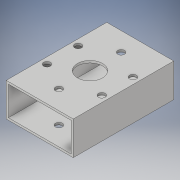
# Autodesk Inventor part: hub attachment
Saved by Autodesk Inventor 2018 (Build 220112000, 112)
## iProperties
Created: 2019-01-30
Part Number: hub attachment
Material: Generic
Document SubType Name: Modeling
Designer: s-4008082
Density: 1 g/cm^3
Appearance: Default
Author: s-4008082
Autodesk Inventor part; units mm, degrees
ref_plane "YZ Plane" through (0, 0, 0) normal (1, 0, 0) x (0, 1, 0)
ref_plane "XZ Plane" through (0, 0, 0) normal (0, 1, 0) x (-1, 0, 0)
ref_plane "XY Plane" through (0, 0, 0) normal (0, 0, 1) x (1, 0, 0)
sketch "Sketch1" plane through (0, 0, 0) normal (0, 0, 1) x (1, 0, 0)
  line L0 (0, 0) -> (50.8, 0)
  line L1 (50.8, 0) -> (50.8, 25.4)
  line L2 (50.8, 25.4) -> (0, 25.4)
  line L3 (0, 25.4) -> (0, 0)
  line L4 (49.149, 23.749) -> (1.651, 23.749)
  line L5 (1.651, 23.749) -> (1.651, 1.651)
  line L6 (1.651, 1.651) -> (49.149, 1.651)
  line L7 (49.149, 1.651) -> (49.149, 23.749)
  line L8 (49.149, 23.749) -> (1.651, 1.651) construction
  line L9 (1.651, 23.749) -> (49.149, 1.651) construction
  point P0 (25.4, 12.7)
  dimension "d0" = 1.651
  dimension "d1" = 25.4
  dimension "d2" = 50.8
  dimension "d3" = 1.651
  dimension "d4" = 1.651
  dimension "d5" = 1.651
  constraints: 20 end point, 4 parallel, 2 horizontal, 2 midpoint, 2 perpendicular
  measures "d0" distance between parallel lines of L2 L4
  measures "d1" distance of L0.end L1.end
  measures "d2" distance of L1.end L2.end
  measures "d3" distance between parallel lines of L1 L7
  measures "d4" distance between parallel lines of L0 L6
  measures "d5" distance between parallel lines of L3 L5
extrude "Extrusion1" add sketch "Sketch1" along normal blind 76.2
sketch "Sketch2" plane through (0, 25.4, 0) normal (0, 1, 0) x (1, 0, 0)
  circle A0 centre (25.4, -38.1) radius 9.525
  line L0 (50.8, 0) -> (50.8, -76.2) projected
  line L1 (50.8, -76.2) -> (0, -76.2) projected
  point P0 (0, 0)
  dimension "d8" = 19.05
  dimension "d9" = 25.4
  dimension "d10" = 38.1
  constraints: 1 centre point
  measures "d8" diameter of A0
  measures "d9" distance from line of L0 A0.centre
  measures "d10" distance from line of L1 A0.centre
extrude "Extrusion2" cut sketch "Sketch2" against normal blind 76.2
sketch "Sketch4" plane through (0, 25.4, 0) normal (0, 1, 0) x (1, 0, 0)
  circle A0 centre (25.1665, -14.2875) radius 2.5797
  circle A1 centre (25.4, -38.1) radius 9.525 projected
  circle A2 centre (25.4, -38.1) radius 23.8136 construction
  circle A3 centre (4.661, -26.396) radius 2.5797
  circle A4 centre (4.8945, -50.2085) radius 2.5797
  circle A5 centre (25.6335, -61.9125) radius 2.5797
  circle A6 centre (46.139, -49.804) radius 2.5797
  circle A7 centre (45.9055, -25.9915) radius 2.5797
  point P0 (0, 0)
  dimension "d31" = 23.8125
  dimension "d32" = 5.1594
  dimension "d35" = 360
  constraints: 6 centre point, 1 coincident, 16 other
  measures "d31" vertical distance of A1.centre A0.centre
  measures "d32" diameter of A0
extrude "Extrusion4" cut sketch "Sketch4" against normal blind 76.2 contours A0 | A3 | A4 | A5 | A6 | A7
equation "\"d3\" = d0"
equation "\"d4\" = d0"
equation "\"d5\" = d0"
body "Solid1"
